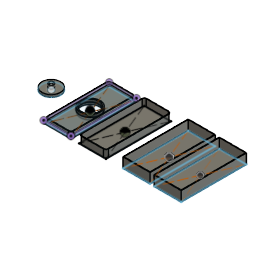
insert (Autodesk Fusion 360 design; units mm, degrees)
Autodesk Fusion 360 part; units mm, degrees
sketch "Sketch4" plane through (0, 10, 0) normal (0, 1, 0) x (-1, 0, 0)
  line L0 (-320, -124) -> (-220, -124)
  line L1 (-220, -124) -> (-220, 124)
  line L2 (-220, 124) -> (-320, 124)
  line L3 (-320, 124) -> (-320, -124)
  line L4 (-320, -124) -> (-220, 124) construction
  line L5 (-220, -124) -> (-320, 124) construction
  line L6 (161.5, 130) -> (-161.5, 130)
  line L7 (-161.5, 130) -> (-161.5, -130)
  line L8 (-161.5, -130) -> (161.5, -130)
  line L9 (161.5, -130) -> (161.5, 130)
  point P0 (-270, 0)
  dimension "d17" = 100
  dimension "d18" = 248
  constraint horizontal L0
  constraint perpendicular L0 L1
  constraint parallel L0 L2
  constraint parallel L1 L3
  constraint coincident L4 P0
  constraint coincident L5 P0
  measures "d17" distance of L1.end L2.end
  measures "d18" distance of L0.end L1.end
sketch "Sketch5" plane through (0, 20, 0) normal (0, 1, 0) x (-1, 0, 0)
sketch "Sketch9" plane through (0, 20, 0) normal (0, 1, 0) x (-1, 0, 0)
sketch "Sketch10" plane through (0, 10, 0) normal (0, 1, 0) x (-1, 0, 0)
sketch "Sketch11" plane through (0, 0, 0) normal (0, 1, 0) x (1, 0, 0)
sketch "Sketch12" plane through (0, 20, 0) normal (0, 1, 0) x (1, 0, 0)
sketch "Sketch14" plane through (0, 0, 0) normal (0, 1, 0) x (1, 0, 0)
sketch "Sketch15" plane through (0, 0, 0) normal (0, 1, 0) x (1, 0, 0)
  line L0 (-160.7431, 132.5987) -> (-51.7431, 132.5987)
  line L1 (-51.7431, 132.5987) -> (-51.7431, -128.8013)
  line L2 (-51.7431, -128.8013) -> (-160.7431, -128.8013)
  line L3 (-160.7431, -128.8013) -> (-160.7431, 132.5987)
  line L4 (-160.7431, 132.5987) -> (-51.7431, -128.8013) construction
  line L5 (-51.7431, 132.5987) -> (-160.7431, -128.8013) construction
  line L6 (-53.7431, 130.5987) -> (-158.7431, 130.5987)
  line L7 (-158.7431, 130.5987) -> (-158.7431, -126.8013)
  line L8 (-158.7431, -126.8013) -> (-53.7431, -126.8013)
  line L9 (-53.7431, -126.8013) -> (-53.7431, 130.5987)
  line L10 (-53.7431, 130.5987) -> (-158.7431, -126.8013) construction
  line L11 (-158.7431, 130.5987) -> (-53.7431, -126.8013) construction
  point P0 (-106.2431, 1.8987)
  point P1 (-106.2431, 1.8987)
  dimension "d42" = 109
  dimension "d43" = 261.4
  dimension "d44" = 105
  dimension "d45" = 257.4
  constraint horizontal L0
  constraint perpendicular L0 L1
  constraint parallel L0 L2
  constraint parallel L1 L3
  constraint coincident L4 P1
  constraint coincident L5 P1
  constraint horizontal L6
  constraint perpendicular L6 L7
  constraint parallel L6 L8
  constraint parallel L7 L9
  constraint coincident L10 P1
  constraint coincident L11 P1
  constraint coincident P1 P0
  measures "d42" distance of L1.end L2.end
  measures "d43" distance of L0.end L1.end
  measures "d44" distance of L7.end L8.end
  measures "d45" distance of L6.end L7.end
extrude "Extrude9" add sketch "Sketch15" along normal blind 10 contours L6 L7 L8 L9 makes body 1
sketch "Sketch16" plane through (0, 0, 0) normal (0, 1, 0) x (1, 0, 0)
sketch "Sketch17" plane through (0, 0, 0) normal (0, 1, 0) x (1, 0, 0)
  line L0 (-35.9, 132.1) -> (73.1, 132.1)
  line L1 (73.1, 132.1) -> (73.1, -129.3)
  line L2 (73.1, -129.3) -> (-35.9, -129.3)
  line L3 (-35.9, -129.3) -> (-35.9, 132.1)
  line L4 (-35.9, 132.1) -> (73.1, -129.3) construction
  line L5 (73.1, 132.1) -> (-35.9, -129.3) construction
  line L6 (71.1, 130.1) -> (-33.9, 130.1)
  line L7 (-33.9, 130.1) -> (-33.9, -127.3)
  line L8 (-33.9, -127.3) -> (71.1, -127.3)
  line L9 (71.1, -127.3) -> (71.1, 130.1)
  line L10 (71.1, 130.1) -> (-33.9, -127.3) construction
  point P0 (18.6, 1.4)
  point P1 (18.6, 1.4)
  dimension "d50" = 109
  dimension "d51" = 261.4
  dimension "d52" = 105
  dimension "d53" = 257.4
  constraint horizontal L0
  constraint perpendicular L0 L1
  constraint parallel L0 L2
  constraint parallel L1 L3
  constraint coincident L4 P1
  constraint coincident L5 P1
  constraint horizontal L6
  constraint perpendicular L6 L7
  constraint parallel L6 L8
  constraint parallel L7 L9
  constraint coincident L10 P1
  constraint coincident P1 P0
  measures "d50" distance of L1.end L2.end
  measures "d51" distance of L0.end L1.end
  measures "d52" distance of L7.end L8.end
  measures "d53" distance of L6.end L7.end
sketch "Sketch35" plane through (0, 0, 0) normal (0, 1, 0) x (1, 0, 0)
  line L0 (-365.7, 130.7) -> (-474.3, 130.7)
  line L1 (-474.3, 130.7) -> (-474.3, -130.7)
  line L2 (-474.3, -130.7) -> (-365.7, -130.7)
  line L3 (-365.7, -130.7) -> (-365.7, 130.7)
  line L4 (-365.7, 130.7) -> (-474.3, -130.7) construction
  line L5 (-474.3, 130.7) -> (-365.7, -130.7) construction
  circle A0 centre (-420, 0) radius 37.5
  point P0 (-420, 0)
  dimension "d73" = 108.6
  dimension "d82" = 75
  dimension "d111" = 261.4
  constraint horizontal L0
  constraint perpendicular L0 L1
  constraint parallel L0 L2
  constraint parallel L1 L3
  constraint coincident L4 P0
  constraint coincident L5 P0
  constraint coincident P0 A0.centre
  measures "d73" distance of L1.end L2.end
  measures "d82" diameter of A0
  measures "d111" distance of L0.end L1.end
sketch "Sketch37" plane through (0, 0, 0) normal (0, 1, 0) x (1, 0, 0)
  line L0 (-368.1512, 128.0997) -> (-471.8512, 128.0997)
  line L1 (-471.8512, 128.0997) -> (-471.8512, -128.1003)
  line L2 (-471.8512, -128.1003) -> (-368.1512, -128.1003)
  line L3 (-368.1512, -128.1003) -> (-368.1512, 128.0997)
  line L4 (-368.1512, 128.0997) -> (-471.8512, -128.1003) construction
  line L5 (-471.8512, 128.0997) -> (-368.1512, -128.1003) construction
  line L6 (-370.1512, 126.0997) -> (-469.8512, 126.0997)
  line L7 (-469.8512, 126.0997) -> (-469.8512, -126.1003)
  line L8 (-469.8512, -126.1003) -> (-370.1512, -126.1003)
  line L9 (-370.1512, -126.1003) -> (-370.1512, 126.0997)
  line L10 (-370.1512, 126.0997) -> (-469.8512, -126.1003) construction
  line L11 (-469.8512, 126.0997) -> (-370.1512, -126.1003) construction
  point P0 (-420.0012, -0.0003)
  point P1 (-420.0012, -0.0003)
  dimension "d76" = 103.7
  dimension "d77" = 256.2
  dimension "d78" = 99.7
  dimension "d79" = 252.2
  constraint horizontal L0
  constraint perpendicular L0 L1
  constraint parallel L0 L2
  constraint parallel L1 L3
  constraint coincident L4 P1
  constraint coincident L5 P1
  constraint horizontal L6
  constraint perpendicular L6 L7
  constraint parallel L6 L8
  constraint parallel L7 L9
  constraint coincident L10 P1
  constraint coincident L11 P1
  constraint coincident P1 P0
  measures "d76" distance of L1.end L2.end
  measures "d77" distance of L0.end L1.end
  measures "d78" distance of L7.end L8.end
  measures "d79" distance of L6.end L7.end
sketch "Sketch38" plane through (0, 0, 0) normal (0, 1, 0) x (1, 0, 0)
extrude "Extrude15" add sketch "Sketch35" along normal blind 10 makes body 2
sketch "Sketch39" plane through (0, 0, 0) normal (0, 1, 0) x (1, 0, 0)
sketch "Sketch40" plane through (0, 0, 0) normal (0, 0, 1) x (1, 0, 0)
sketch "Sketch41" plane through (0, 0, 0) normal (0, 1, 0) x (1, 0, 0)
sketch "Sketch42" plane through (0, 0, 0) normal (0, 1, 0) x (1, 0, 0)
  line L0 (-227.9, 128.7) -> (-332.5, 128.7)
  line L1 (-332.5, 128.7) -> (-332.5, -128.7)
  line L2 (-332.5, -128.7) -> (-227.9, -128.7)
  line L3 (-227.9, -128.7) -> (-227.9, 128.7)
  line L4 (-227.9, 128.7) -> (-332.5, -128.7) construction
  line L5 (-332.5, 128.7) -> (-227.9, -128.7) construction
  line L6 (-225.9, 130.7) -> (-334.5, 130.7)
  line L7 (-334.5, 130.7) -> (-334.5, -130.7)
  line L8 (-334.5, -130.7) -> (-225.9, -130.7)
  line L9 (-225.9, -130.7) -> (-225.9, 130.7)
  line L10 (-225.9, 130.7) -> (-334.5, -130.7) construction
  line L11 (-334.5, 130.7) -> (-225.9, -130.7) construction
  point P0 (-280.2, 0)
  point P1 (-280.2, 0)
  dimension "d85" = 104.6
  dimension "d86" = 257.4
  dimension "d196" = 108.6
  dimension "d197" = 261.4
  constraint horizontal L0
  constraint perpendicular L0 L1
  constraint parallel L0 L2
  constraint parallel L1 L3
  constraint coincident L4 P1
  constraint coincident L5 P1
  constraint horizontal L6
  constraint perpendicular L6 L7
  constraint parallel L6 L8
  constraint parallel L7 L9
  constraint coincident L10 P1
  constraint coincident L11 P1
  constraint coincident P1 P0
  measures "d85" distance of L1.end L2.end
  measures "d86" distance of L0.end L1.end
  measures "d196" distance of L7.end L8.end
  measures "d197" distance of L6.end L7.end
sketch "Sketch43" plane through (0, 0, 0) normal (0, 1, 0) x (1, 0, 0)
sketch "Sketch44" plane through (0, 0, 0) normal (0, 1, 0) x (1, 0, 0)
sketch "Sketch45" plane through (0, 10, 0) normal (0, 1, 0) x (-1, 0, 0)
  circle A0 centre (420, 0) radius 37.5
  circle A1 centre (420, 0) radius 40
  circle A2 centre (420, 0) radius 35
  line L0 (365.7, 130.7) -> (365.7, -130.7)
  line L1 (365.7, -130.7) -> (474.3, -130.7)
  line L2 (474.3, -130.7) -> (474.3, 130.7)
  line L3 (474.3, 130.7) -> (365.7, 130.7)
  dimension "d91" = 80
  dimension "d92" = 70
  constraint concentric A0 A1
  constraint concentric A0 A2
  measures "d91" diameter of A1
  measures "d92" diameter of A2
extrude "Extrude18" add sketch "Sketch45" along normal blind 5 contours A0 | A1 bodies 2
sketch "Sketch46" plane through (0, 0, 0) normal (0, 0, 1) x (1, 0, 0)
sketch "Sketch47" plane through (0, 0, 0) normal (0, 1, 0) x (1, 0, 0)
sketch "Sketch48" plane through (0, 0, 0) normal (0, 1, 0) x (1, 0, 0)
  circle A0 centre (-575, 0) radius 37.2
  circle A1 centre (-575, 0) radius 10
  dimension "d95" = 74.4
  dimension "d96" = 20
  constraint concentric A0 A1
  measures "d95" diameter of A0
  measures "d96" diameter of A1
extrude "Extrude19" add sketch "Sketch48" along normal blind 25 separate body contours A1 makes body 3
sketch "Sketch49" plane through (0, 0, 0) normal (0, 1, 0) x (1, 0, 0)
extrude "Extrude20" add sketch "Sketch48" along normal blind 9.6 bodies 3
fillet "Fillet1" radius 3 1 edges at (-584.3233, 25, 3.6162) on bodies 3
extrude "Extrude26" add sketch "Sketch42" along normal blind 10 contours L0 L1 L2 L3 makes body 4
extrude "Extrude28" cut 1 faces at (-123.7431, 10, 41.0013) along direction (0, -1, 0) blind 8 on bodies 1 bodies 1
extrude "Extrude29" cut 1 faces at (-297.6333, 10, -42.9) along direction (0, -1, 0) blind 8 on bodies 4 bodies 4
extrude "Extrude30" cut 1 faces at (-420.9964, 10, 100.4294) along direction (0, -1, 0) blind 8 on bodies 2 bodies 2
extrude "Extrude31" add sketch "Sketch15" along normal blind 40 bodies 1
fillet "Fillet38" radius 10 1 edges at (-158.7431, 21, 126.8013) on bodies 1
fillet "Fillet39" radius 10 1 edges at (-53.7431, 21, 126.8013) on bodies 1
fillet "Fillet40" radius 10 1 edges at (-53.7431, 21, -130.5987) on bodies 1
fillet "Fillet41" radius 10 1 edges at (-158.7431, 21, -130.5987) on bodies 1
fillet "Fillet42" radius 10 1 edges at (-51.7431, 20, 128.8013) on bodies 1
fillet "Fillet43" radius 10 1 edges at (-160.7431, 20, 128.8013) on bodies 1
fillet "Fillet44" radius 10 1 edges at (-160.7431, 20, -132.5987) on bodies 1
fillet "Fillet45" radius 10 1 edges at (-51.7431, 20, -132.5987) on bodies 1
extrude "Extrude33" add sketch "Sketch42" along normal blind 30 bodies 4
fillet "Fillet54" radius 8 1 edges at (-332.5, 16, 128.7) on bodies 4
fillet "Fillet55" radius 8 1 edges at (-332.5, 16, -128.7) on bodies 4
fillet "Fillet56" radius 8 1 edges at (-227.9, 16, -128.7) on bodies 4
fillet "Fillet57" radius 8 1 edges at (-227.9, 16, 128.7) on bodies 4
fillet "Fillet58" radius 10 1 edges at (-225.9, 15, 130.7) on bodies 4
fillet "Fillet59" radius 10 1 edges at (-334.5, 15, 130.7) on bodies 4
fillet "Fillet60" radius 10 1 edges at (-334.5, 15, -130.7) on bodies 4
fillet "Fillet61" radius 10 1 edges at (-225.9, 15, -130.7) on bodies 4
extrude "Extrude34" add sketch "Sketch35" along normal blind 10 separate body makes body 5
extrude "Extrude36" add sketch "Sketch45" along normal blind 10 contours A1 bodies 5
extrude "Extrude37" add sketch "Sketch45" along normal blind 10 contours A0 bodies 5
form "Form1" [no effect]
extrude "Extrude38" add sketch "Sketch37" along normal blind 20 separate body makes body 6
fillet "Fillet64" radius 8 1 edges at (-469.8512, 10, 126.1003) on bodies 6
fillet "Fillet65" radius 8 1 edges at (-469.8512, 10, -126.0997) on bodies 6
fillet "Fillet66" radius 8 1 edges at (-370.1512, 10, -126.0997) on bodies 6
fillet "Fillet67" radius 8 1 edges at (-370.1512, 10, 126.1003) on bodies 6
fillet "Fillet68" radius 10 1 edges at (-368.1512, 10, 128.1003) on bodies 6
fillet "Fillet69" radius 10 1 edges at (-471.8512, 10, 128.1003) on bodies 6
fillet "Fillet70" radius 10 1 edges at (-471.8512, 10, -128.0997) on bodies 6
fillet "Fillet71" radius 10 1 edges at (-474.3, 5, -130.7) on bodies 5
fillet "Fillet72" radius 10 1 edges at (-474.3, 5, 130.7) on bodies 5
fillet "Fillet73" radius 10 1 edges at (-365.7, 5, 130.7) on bodies 5
fillet "Fillet74" radius 10 1 edges at (-368.1512, 10, -128.0997) on bodies 6
fillet "Fillet75" radius 10 1 edges at (-365.7, 5, -130.7) on bodies 5
combine "Combine1" operation add target body 6 tool bodies 5
extrude "Extrude39" add sketch "Sketch17" along normal blind 40 separate body makes body 7
extrude "Extrude40" add sketch "Sketch17" along normal blind 2 contours L6 L7 L8 L9 bodies 7
fillet "Fillet76" radius 20 1 edges at (-33.9, 21, 127.3) on bodies 7
fillet "Fillet77" radius 20 1 edges at (-33.9, 21, -130.1) on bodies 7
fillet "Fillet78" radius 20 1 edges at (71.1, 21, -130.1) on bodies 7
fillet "Fillet79" radius 20 1 edges at (71.1, 21, 127.3) on bodies 7
fillet "Fillet80" radius 20 1 edges at (-35.9, 20, -132.1) on bodies 7
fillet "Fillet81" radius 20 1 edges at (73.1, 20, -132.1) on bodies 7
fillet "Fillet82" radius 20 1 edges at (73.1, 20, 129.3) on bodies 7
fillet "Fillet83" radius 20 1 edges at (-35.9, 20, 129.3) on bodies 7
delete_face "DeleteFace3" 1 faces at (-31.6211, 26.6667, 121.6632) on bodies 7
delete_face "DeleteFace4" 1 faces at (55.0011, 26.6667, 129.2094) on bodies 7
delete_face "DeleteFace5" 1 faces at (-28.3747, 14.6667, 121.1016) on bodies 7
delete_face "DeleteFace6" 1 faces at (70.5362, 14.6667, 112.0152) on bodies 7
delete_face "DeleteFace7" 1 faces at (62.2645, 13.3333, -129.8767) on bodies 7
delete_face "DeleteFace8" 1 faces at (-35.8094, 13.3333, -114.0011) on bodies 7
delete_face "DeleteFace9" 1 faces at (-51.7544, 13.3333, -123.0745) on bodies 1
delete_face "DeleteFace10" 1 faces at (-152.6356, 13.3333, -132.418) on bodies 1
delete_face "DeleteFace11" 1 faces at (-151.1007, 14.6667, -130.3168) on bodies 1
delete_face "DeleteFace12" 1 faces at (-53.7884, 14.6667, -121.5492) on bodies 1
delete_face "DeleteFace13" 1 faces at (70, 14.6667, -116.6414) on bodies 7
delete_face "DeleteFace14" 1 faces at (-33.3362, 27.3333, -114.8152) on bodies 7
delete_face "DeleteFace15" 1 faces at (-52.025, 26.6667, 121.1589) on bodies 1
delete_face "DeleteFace16" 1 faces at (-152.6356, 13.3333, 128.6206) on bodies 1
delete_face "DeleteFace17" 1 faces at (-54.4594, 14.6667, 120.5179) on bodies 1
delete_face "DeleteFace18" 1 faces at (-158.6978, 14.6667, 117.7519) on bodies 1
hidden bodies 2
equation "d76 = 104 mm - 0.3 mm"
equation "d77 = 257.4 mm - 1.2 mm"
equation "d78 = 100 mm - 0.3 mm"
equation "d79 = 253.4 mm - 1.2 mm"
